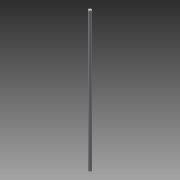
# Autodesk Inventor part: Shorter Shaft
Saved by Autodesk Inventor 2014 SP1 (Build 180222100, 222)
## iProperties
Created: 2013-01-18
Part Number: Shorter Shaft
Material: Aluminum 6061
Document SubType Name: Modeling
Designer: actoennies
Mass: 102.758 g
Surface Area: 160.808 cm^2
Volume: 37.9182 cm^3
Density: 2.71 g/cm^3
Appearance: Aluminum - Flat
Author: actoennies
Autodesk Inventor part; units mm, degrees
ref_plane "YZ Plane" through (0, 0, 0) normal (1, 0, 0) x (0, 1, 0)
ref_plane "XZ Plane" through (0, 0, 0) normal (0, 1, 0) x (-1, 0, 0)
ref_plane "XY Plane" through (0, 0, 0) normal (0, 0, 1) x (1, 0, 0)
sketch "Sketch1" plane through (0, 0, 0) normal (0, 1, 0) x (-1, 0, 0)
  line L0 (-5.4993, 0) -> (-2.7496, 4.7625)
  line L1 (-2.7496, 4.7625) -> (2.7496, 4.7625)
  line L2 (2.7496, 4.7625) -> (5.4993, 0)
  line L3 (5.4993, 0) -> (2.7496, -4.7625)
  line L4 (2.7496, -4.7625) -> (-2.7496, -4.7625)
  line L5 (-2.7496, -4.7625) -> (-5.4993, 0)
  point P0 (0, 0)
  point P1 (0, 0)
  dimension "d0" = 9.525
  constraints: 12 end point, 1 coincident, 13 other
  measures "d0" distance between parallel lines of L4 L1
extrude "Extrusion1" add sketch "Sketch1" along normal blind 482.6
body "Solid1"
